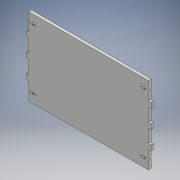
# Autodesk Inventor part: pinball-case-back
Saved by Autodesk Inventor 2017 (Build 210142000, 142)
## iProperties
Created: 2017-03-05
Part Number: pinball-case-back
Material: Generic
Document SubType Name: Modeling
Designer: John
Density: 1 g/cm^3
Appearance: Default
Author: John
Autodesk Inventor part; units mm, degrees
ref_plane "YZ Plane" through (0, 0, 0) normal (1, 0, 0) x (0, 1, 0)
ref_plane "XZ Plane" through (0, 0, 0) normal (0, 1, 0) x (-1, 0, 0)
ref_plane "XY Plane" through (0, 0, 0) normal (0, 0, 1) x (1, 0, 0)
sketch "Sketch1" plane through (0, 0, 0) normal (0, 1, 0) x (-1, 0, 0)
  line L0 (0, 0) -> (271, 0)
  line L1 (271, 0) -> (271, 176)
  line L2 (271, 176) -> (0, 176)
  line L3 (0, 176) -> (0, 0)
  line L4 (-6, 136) -> (0, 136)
  line L5 (0, 136) -> (0, 124)
  line L6 (0, 124) -> (-6, 124)
  line L7 (-6, 124) -> (-6, 136)
  line L8 (-6, 94) -> (0, 94)
  line L9 (0, 94) -> (0, 82)
  line L10 (0, 82) -> (-6, 82)
  line L11 (-6, 82) -> (-6, 94)
  line L12 (-6, 52) -> (0, 52)
  line L13 (0, 52) -> (0, 40)
  line L14 (0, 40) -> (-6, 40)
  line L15 (-6, 40) -> (-6, 52)
  circle A0 centre (-3, 156) radius 1.25
  circle A1 centre (-3, 20) radius 1.25
  line L16 (-3, 40) -> (-3, 20) construction
  line L17 (135.5, 176) -> (135.5, 0) construction
  line L18 (277, 40) -> (277, 52)
  line L19 (271, 40) -> (277, 40)
  line L20 (271, 52) -> (271, 40)
  line L21 (277, 52) -> (271, 52)
  line L22 (271, 82) -> (277, 82)
  line L23 (277, 94) -> (271, 94)
  line L24 (271, 94) -> (271, 82)
  line L25 (277, 82) -> (277, 94)
  line L26 (271, 124) -> (277, 124)
  line L27 (271, 136) -> (271, 124)
  line L28 (277, 136) -> (271, 136)
  line L29 (277, 124) -> (277, 136)
  point P0 (274, 40)
  dimension "d0" = 271
  dimension "d2" = 6
  dimension "d3" = 12
  dimension "d4" = 30
  dimension "d5" = 30
  dimension "d6" = 2.5
  dimension "d7" = 2.5
  dimension "d8" = 20
  dimension "d9" = 20
  dimension "d10" = 20
  dimension "d13" = 20
  constraints: 60 end point, 13 symmetric about line, 8 parallel, 4 horizontal, 4 perpendicular, 4 point on line, 3 equal length, 3 midpoint, 2 centre point, 2 collinear, 1 vertical
  measures "d0" distance of L2.end L1.end
  measures "d2" distance of L6.start L6.end
  measures "d3" distance of L5.start L6.start
  measures "d4" distance between parallel lines of L6 L8
  measures "d5" distance between parallel lines of L12 L10
  measures "d6" diameter of A0
  measures "d7" diameter of A1
  measures "d8" distance from line of L16.end L14
  measures "d9" distance from line of L4 A0.centre
  measures "d10" distance from line of L0 L16.end
  measures "d13" distance from line of A0.centre L2
extrude "Extrusion1" add sketch "Sketch1" along normal blind 6 contours L3 L2 L1 L0 | L14 L15 L12 L3 | L1 L21 L18 L19 | L10 L11 L8 L3 | L1 L23 L25 L22 | L6 L7 L4 L3 | L1 L28 L29 L26
sketch "Sketch2" plane through (0, 6, 0) normal (0, 1, 0) x (1, 0, 0)
  line L0 (0, -40) -> (0, 0) projected
  line L1 (0, -18.75) -> (-8, -18.75)
  line L2 (-17, -18.75) -> (-17, -21.25)
  line L3 (-17, -21.25) -> (-10.3, -21.25)
  line L4 (0, -21.25) -> (0, -18.75)
  line L5 (0, 0) -> (-271, 0) projected
  line L6 (-8, -22.7) -> (-10.3, -22.7)
  line L7 (-10.3, -22.7) -> (-10.3, -21.25)
  line L8 (-10.3, -17.3) -> (-8, -17.3)
  line L9 (-8, -17.3) -> (-8, -18.75)
  line L10 (-8, -21.25) -> (-8, -22.7)
  line L11 (-8, -18.75) -> (-8, -21.25) construction
  line L12 (-10.3, -21.25) -> (-10.3, -18.75) construction
  line L13 (-10.3, -18.75) -> (-10.3, -17.3)
  line L14 (-8, -21.25) -> (0, -21.25)
  line L15 (-10.3, -21.25) -> (-8, -21.25) construction
  line L16 (-8, -18.75) -> (-10.3, -18.75) construction
  line L17 (-10.3, -18.75) -> (-17, -18.75)
  line L18 (0, -154.75) -> (-8, -154.75)
  line L19 (-17, -154.75) -> (-17, -157.25)
  line L20 (-17, -157.25) -> (-10.3, -157.25)
  line L21 (0, -157.25) -> (0, -154.75)
  line L22 (-8, -158.7) -> (-10.3, -158.7)
  line L23 (-10.3, -158.7) -> (-10.3, -157.25)
  line L24 (-10.3, -153.3) -> (-8, -153.3)
  line L25 (-8, -153.3) -> (-8, -154.75)
  line L26 (-8, -157.25) -> (-8, -158.7)
  line L27 (-8, -154.75) -> (-8, -157.25) construction
  line L28 (-10.3, -157.25) -> (-10.3, -154.75) construction
  line L29 (-10.3, -154.75) -> (-10.3, -153.3)
  line L30 (-8, -157.25) -> (0, -157.25)
  line L31 (-10.3, -157.25) -> (-8, -157.25) construction
  line L32 (-8, -154.75) -> (-10.3, -154.75) construction
  line L33 (-10.3, -154.75) -> (-17, -154.75)
  line L34 (0, -176) -> (0, -136) projected
  line L35 (-271, -176) -> (0, -176) projected
  line L36 (-135.5, -176) -> (-135.5, 0) construction
  line L37 (-271, -18.75) -> (-263, -18.75)
  line L38 (-254, -18.75) -> (-254, -21.25)
  line L39 (-254, -21.25) -> (-260.7, -21.25)
  line L40 (-271, -21.25) -> (-271, -18.75)
  line L41 (-263, -22.7) -> (-260.7, -22.7)
  line L42 (-260.7, -22.7) -> (-260.7, -21.25)
  line L43 (-260.7, -17.3) -> (-263, -17.3)
  line L44 (-263, -17.3) -> (-263, -18.75)
  line L45 (-263, -21.25) -> (-263, -22.7)
  line L46 (-263, -18.75) -> (-263, -21.25) construction
  line L47 (-260.7, -21.25) -> (-260.7, -18.75) construction
  line L48 (-260.7, -18.75) -> (-260.7, -17.3)
  line L49 (-263, -21.25) -> (-271, -21.25)
  line L50 (-260.7, -21.25) -> (-263, -21.25) construction
  line L51 (-263, -18.75) -> (-260.7, -18.75) construction
  line L52 (-260.7, -18.75) -> (-254, -18.75)
  line L53 (-260.7, -158.7) -> (-260.7, -157.25)
  line L54 (-260.7, -157.25) -> (-263, -157.25) construction
  line L55 (-260.7, -157.25) -> (-260.7, -154.75) construction
  line L56 (-263, -157.25) -> (-263, -158.7)
  line L57 (-263, -158.7) -> (-260.7, -158.7)
  line L58 (-263, -154.75) -> (-260.7, -154.75) construction
  line L59 (-263, -154.75) -> (-263, -157.25) construction
  line L60 (-260.7, -154.75) -> (-260.7, -153.3)
  line L61 (-260.7, -153.3) -> (-263, -153.3)
  line L62 (-263, -153.3) -> (-263, -154.75)
  line L63 (-254, -157.25) -> (-260.7, -157.25)
  line L64 (-260.7, -154.75) -> (-254, -154.75)
  line L65 (-254, -154.75) -> (-254, -157.25)
  line L66 (-263, -157.25) -> (-271, -157.25)
  line L67 (-271, -154.75) -> (-263, -154.75)
  line L68 (-271, -157.25) -> (-271, -154.75)
  point P0 (-271, -40)
  point P1 (-271, -136)
  dimension "d14" = 17
  dimension "d15" = 2.5
  dimension "d16" = 18.75
  dimension "d19" = 2.3
  dimension "d20" = 5.4
  dimension "d21" = 8
  dimension "d22" = 17
  dimension "d23" = 2.5
  dimension "d24" = 2.3
  dimension "d25" = 5.4
  dimension "d26" = 18.75
  constraints: 130 end point, 40 parallel, 26 symmetric about line, 12 perpendicular, 8 horizontal, 5 point on line, 3 collinear, 2 midpoint
  measures "d14" distance of L4.start L2.end
  measures "d15" distance of L2.end L2.start
  measures "d16" distance between parallel lines of L5 L1
  measures "d19" distance of L8.start L8.end
  measures "d20" distance of L6.end L8.start
  measures "d21" distance between parallel lines of L0 L10
  measures "d22" distance of L30.end L20.start
  measures "d23" distance of L20.start L33.end
  measures "d24" distance of L29.end L24.end
  measures "d25" distance of L23.start L29.end
  measures "d26" distance between parallel lines of L30 L35
extrude "Extrusion2" cut sketch "Sketch2" against normal through all
equation "\"d5\" = d4"
equation "\"d6\" = d7"
equation "\"d9\" = d8"
equation "\"d26\" = d16"
body "Solid1"
